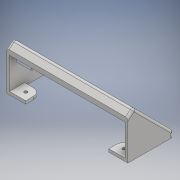
# Autodesk Inventor part: holder-LCD-screen
Saved by Autodesk Inventor 2018 (Build 220112000, 112)
## iProperties
Created: 2017-11-05
Part Number: holder-LCD-screen
Material: Generic
Document SubType Name: Modeling
Designer: Jurjen
Density: 1 g/cm^3
Appearance: Default
Author: Jurjen
Autodesk Inventor part; units mm, degrees
ref_plane "YZ Plane" through (0, 0, 0) normal (1, 0, 0) x (0, 1, 0)
ref_plane "XZ Plane" through (0, 0, 0) normal (0, 1, 0) x (-1, 0, 0)
ref_plane "XY Plane" through (0, 0, 0) normal (0, 0, 1) x (1, 0, 0)
sketch "Sketch1" plane through (0, 0, 0) normal (1, 0, 0) x (0, 1, 0)
  line L0 (-30, 25.7931) -> (-30, -25.7931)
  line L1 (30, -18.7931) -> (-21.6188, 32.8257)
  line L2 (-21.6188, 32.8257) -> (-30, 25.7931)
  line L3 (30, -18.7931) -> (30, -25.7931)
  line L4 (30, -25.7931) -> (-30, -25.7931)
  point P0 (0, 0)
  point P1 (-30, 0)
  point P2 (0, -25.7931)
  point P3 (-30, 0)
  dimension "d3" = 50
  dimension "d4" = 73
  dimension "d8" = 60
  dimension "d9" = 45
  dimension "d10" = 7
  constraints: 10 end point, 3 midpoint, 2 horizontal alignment, 2 vertical, 1 perpendicular, 1 vertical alignment
  measures "d3" angle of L2 L0
  measures "d4" distance of L1.start L1.end
  measures "d8" distance of L3.end L0.end
  measures "d9" angle of L4 L1
  measures "d10" distance of L1.start L3.end
extrude "Extrusion1" add sketch "Sketch1" along normal mid plane 160
sketch "Sketch2" plane through (-80, -21.6188, 32.8257) normal (0, 0.7071068, 0.7071068) x (1, 0, 0)
  line L0 (3.5, 69.5) -> (156.5, 69.5)
  line L1 (156.5, 69.5) -> (156.5, 3.5)
  line L2 (156.5, 3.5) -> (3.5, 3.5)
  line L3 (3.5, 3.5) -> (3.5, 69.5)
  line L4 (0, 0) -> (0, 73) projected
  line L5 (0, 0) -> (160, 0) projected
  line L6 (0, 73) -> (160, 73) projected
  line L7 (160, 73) -> (160, 0) projected
  point P0 (80, 38.4981)
  dimension "d11" = 3.5
  dimension "d12" = 3.5
  dimension "d13" = 3.5
  dimension "d14" = 3.5
  constraints: 8 end point, 2 parallel, 1 horizontal, 1 perpendicular
  measures "d11" distance between parallel lines of L4 L3
  measures "d12" distance between parallel lines of L5 L2
  measures "d13" distance between parallel lines of L6 L0
  measures "d14" distance between parallel lines of L7 L1
extrude "Extrusion2" cut sketch "Sketch2" against normal up to next contours L0 L1 L2 L3
sketch "Sketch3" plane through (-80, -21.6188, 32.8257) normal (0, 0.7071068, 0.7071068) x (1, 0, 0)
  line L0 (3.5, 3.5) -> (3.5, 69.5) projected
  line L1 (3.5, 69.5) -> (156.5, 69.5) projected
  line L2 (156.5, 69.5) -> (156.5, 3.5) projected
  line L3 (156.5, 3.5) -> (3.5, 3.5) projected
  line L4 (0, 0) -> (160, 0) projected
  line L5 (160, 73) -> (160, 0) projected
  line L6 (0, 73) -> (160, 73) projected
  line L7 (0, 0) -> (0, 73) projected
  line L8 (3.5, 69.5) -> (156.5, 69.5)
  line L9 (156.5, 69.5) -> (156.5, 3.5)
  line L10 (156.5, 3.5) -> (3.5, 3.5)
  line L11 (3.5, 3.5) -> (3.5, 69.5)
  line L12 (18.7, 55) -> (117.2, 55)
  line L13 (117.2, 55) -> (117.2, 14.5)
  line L14 (117.2, 14.5) -> (18.7, 14.5)
  line L15 (18.7, 14.5) -> (18.7, 55)
  circle A0 centre (143.6, 37.2) radius 6.25
  circle A1 centre (143.1, 56.2) radius 6.5
  point P0 (80, 38.4981)
  dimension "d17" = 98.5
  dimension "d18" = 40.5
  dimension "d19" = 26.4
  dimension "d20" = 12.5
  dimension "d21" = 22.7
  dimension "d22" = 15.2
  dimension "d23" = 11
  dimension "d67" = 13
  dimension "d69" = 0.5
  dimension "d70" = 19
  constraints: 16 end point, 4 parallel, 2 centre point, 2 horizontal, 2 perpendicular
  measures "d17" distance between parallel lines of L13 L15
  measures "d18" distance between parallel lines of L14 L12
  measures "d19" distance from line of L13 A0.centre
  measures "d20" diameter of A0
  measures "d21" distance from line of A0.centre L14
  measures "d22" distance between parallel lines of L0 L15
  measures "d23" distance between parallel lines of L3 L14
  measures "d67" diameter of A1
  measures "d69" horizontal distance of A0.centre A1.centre
  measures "d70" vertical distance of A0.centre A1.centre
extrude "Extrusion3" add sketch "Sketch3" against normal blind 3 contours L0 L1 L2 L3
fillet "Fillet1" radius 3 8 edges at (0, -21.6188, 32.8257) (-80, 4.1906, 7.0163) (-80, -25.8094, 29.3094) (80, -25.8094, 29.3094) (80, 4.1906, 7.0163) (0, 30, -18.7931) (-80, 30, -22.2931) (80, 30, -22.2931)
sketch "Sketch4" plane through (76.5, 18.0503, -25.7931) normal (0, 0, -1) x (-1, 0, 0)
  line L0 (137.8, -2.8995) -> (137.8, -31.5373) projected
  line L1 (137.8, -31.5373) -> (39.3, -31.5373) projected
  line L2 (39.3, -31.5373) -> (39.3, -2.8995) projected
  line L3 (39.3, -2.8995) -> (137.8, -2.8995) projected
  ellipse E0 centre (12.9, -15.486) end of major axis (19.15, -15.486) minor radius 4.4194 projected
  line L4 (153, 7.3536) -> (153, -39.3155) projected
  line L5 (0, 7.3536) -> (153, 7.3536) projected
  line L6 (0, -39.3155) -> (0, 7.3536) projected
  line L7 (153, -39.3155) -> (0, -39.3155) projected
  line L8 (153, 0) -> (153, -48.0503) projected
  line L9 (0, 7.3536) -> (153, 7.3536)
  line L10 (153, 7.3536) -> (153, 0)
  line L11 (153, 0) -> (0, 0)
  line L12 (0, 0) -> (0, 7.3536)
  point P0 (76.5, -18.0503)
  constraints: 8 end point, 2 parallel, 1 horizontal, 1 perpendicular, 1 other
extrude "Extrusion4" cut sketch "Sketch4" against normal up to next contours L4 L11 L6 L5
sketch "Sketch5" plane through (-80, 0, 0) normal (-1, 0, 0) x (0, 0, 1)
  line L0 (-13.3123, -0.2295) -> (7.9009, -21.4427)
  line L1 (7.9009, -21.4427) -> (12.1436, -17.2001)
  line L2 (12.1436, -17.2001) -> (-9.0696, 4.0131)
  line L3 (-9.0696, 4.0131) -> (-13.3123, -0.2295)
  line L4 (-20.0357, 27) -> (28.7606, -21.7963) projected
  line L5 (28.2295, -21.2652) -> (-18.4395, 25.4038) projected
  line L6 (-18.4395, 25.4038) -> (28.2295, -21.2652) projected
  line L7 (8.8195, -1.8552) -> (-0.0194, 6.9837) projected
  line L8 (-8.1865, 15.1508) -> (20.4514, -13.4871) projected
  line L9 (20.4514, -13.4871) -> (-8.1865, 15.1508) projected
  point P0 (0, 0)
  dimension "d35" = 30
  dimension "d36" = 6
  dimension "d39" = 14.5
  dimension "d40" = 15
  constraints: 8 end point, 3 perpendicular, 1 parallel
  measures "d35" distance of L1.end L2.end
  measures "d36" distance between parallel lines of L2 L0
  measures "d39" distance between parallel lines of L4 L0
  measures "d40" distance from line of L4.end L1
extrude "Extrusion5" cut sketch "Sketch5" against normal up to next
sketch "Sketch6" plane through (-77, -19.675, 30.8819) normal (0, 0.7071068, 0.7071068) x (1, 0, 0)
  circle A0 centre (4.1, 61.451) radius 1.6
  circle A1 centre (4.1, 11.951) radius 1.6
  circle A2 centre (148.6, 61.451) radius 1.6
  circle A3 centre (148.6, 11.951) radius 1.6
  line L0 (0.5, 71.9508) -> (0.5, 32.7743) projected
  line L1 (0.5, 0.751) -> (153.5, 0.751) projected
  circle A4 centre (5.7, 61.451) radius 1.6
  circle A5 centre (5.7, 11.951) radius 1.6
  circle A6 centre (147, 11.951) radius 1.6
  circle A7 centre (147, 61.451) radius 1.6
  line L2 (147, 63.051) -> (148.6, 63.051)
  line L3 (147, 59.851) -> (148.6, 59.851)
  line L4 (4.1, 63.051) -> (5.7, 63.051)
  line L5 (4.1, 59.851) -> (5.7, 59.851)
  line L6 (4.1, 13.551) -> (5.7, 13.551)
  line L7 (5.7, 10.351) -> (4.1, 10.351)
  line L8 (147, 13.551) -> (148.6, 13.551)
  line L9 (147, 10.351) -> (148.6, 10.351)
  point P0 (77, 35.7491)
  dimension "d41" = 3.2
  dimension "d42" = 144.5
  dimension "d43" = 49.5
  dimension "d44" = 3.6
  dimension "d45" = 11.2
  constraints: 20 point on circle, 16 end point, 9 tangent, 8 centre point, 7 equal radius, 5 parallel, 3 point on line, 2 horizontal, 2 horizontal alignment, 2 vertical alignment
  measures "d41" diameter of A0
  measures "d42" distance of A2.centre A0.centre
  measures "d43" distance of A0.centre A1.centre
  measures "d44" distance from line of A0.centre L0
  measures "d45" distance from line of A1.centre L1
extrude "Extrusion6" cut sketch "Sketch6" against normal up to next contours A0 A4 | A0 A4 | A1 A5 | A1 A5 | A2 A7 | A2 A7 L2 | L3 A7 A2 | A7 A2 | A2 A7 | A3 A6 | A3 A6 L8 | L9 A6 A3 | A6 A3 | A3 A6 picked at (3.0447, 61.5129) picked at (4.6405, 61.451) picked at (3.0447, 12.0129) picked at (4.6405, 11.951)
chamfer "Chamfer1" distance 2 angle 45 4 edges at (-80, -10.8361, -2.7057) (-80, 1.8918, -11.191) (-80, -6.5935, 1.537) (-80, -19.3214, 10.0222)
sketch "Sketch7" plane through (77, 30, -25.7931) normal (0, 0, -1) x (-1, 0, 0)
  line L0 (157, -51.7963) -> (157, -60) projected
  line L1 (157, -60) -> (132, -60)
  line L2 (132, -60) -> (132, -40)
  line L3 (132, -40) -> (157, -40)
  line L4 (157, -40) -> (157, -60)
  point P0 (77, -30)
  dimension "d51" = 25
  dimension "d52" = 20
  constraints: 8 end point, 2 parallel, 1 horizontal, 1 perpendicular
  measures "d51" distance between parallel lines of L4 L2
  measures "d52" distance between parallel lines of L1 L3
extrude "Extrusion7" add sketch "Sketch7" against normal blind 4
sketch "Sketch8" plane through (77, 30, -25.7931) normal (0, 0, -1) x (-1, 0, 0)
  circle A0 centre (142, -50) radius 2.1
  line L0 (157, -60) -> (132, -60) projected
  line L1 (132, -60) -> (132, -40) projected
  point P0 (77, -30)
  dimension "d55" = 10
  dimension "d56" = 10
  dimension "d57" = 4.2
  constraints: 1 centre point
  measures "d55" distance from line of L0 A0.centre
  measures "d56" distance from line of L1 A0.centre
  measures "d57" diameter of A0
fillet "Fillet2" radius 10 1 edges at (-55, -10, -23.7931)
extrude "Extrusion8" cut sketch "Sketch8" against normal up to next
mirror "Mirror1" about plane through (0, 0, 0) normal (1, 0, 0) of "Extrusion7", "Fillet2", "Extrusion8"
sketch "Sketch9" plane through (-77, -19.675, 30.8819) normal (0, 0.7071068, 0.7071068) x (1, 0, 0)
  line L0 (15.7, 64.6999) -> (54.0715, 64.6999) construction
  line L1 (54.0715, 64.6999) -> (54.0715, 56.5594) construction
  line L2 (54.0715, 56.5594) -> (15.7, 56.5594) construction
  line L3 (15.7, 56.5594) -> (15.7, 64.6999) construction
  line L4 (15.7, 52.251) -> (114.2, 52.251) projected
  line L5 (0, 69.0084) -> (154, 69.0084) projected
  line L6 (114.2, 52.251) -> (114.2, 69.0084) construction
  line L7 (21.5476, 60.6463) -> (20.0354, 60.3719)
  spline S0 degree 2 poles (20.0354, 60.3719) (19.9622, 60.8231) (19.4195, 61.2804) (18.9866, 61.2804) knots 0 0 0 1 2 2 2
  spline S1 degree 2 poles (18.9866, 61.2804) (18.4195, 61.2804) (17.7366, 60.4877) (17.7366, 59.5609) knots 0 0 0 1 2 2 2
  spline S2 degree 2 poles (17.7366, 59.5609) (17.7366, 58.5304) (18.4317, 57.6829) (19.011, 57.6829) knots 0 0 0 1 2 2 2
  spline S3 degree 2 poles (19.011, 57.6829) (19.45, 57.6829) (20.0049, 58.1829) (20.1207, 58.7865) knots 0 0 0 1 2 2 2
  line L8 (20.1207, 58.7865) -> (21.6268, 58.5304)
  spline S4 degree 2 poles (21.6268, 58.5304) (21.3951, 57.4938) (20.0598, 56.4329) (18.9439, 56.4329) knots 0 0 0 1 2 2 2
  spline S5 degree 2 poles (18.9439, 56.4329) (17.6756, 56.4329) (16.1634, 58.0365) (16.1634, 59.4572) knots 0 0 0 1 2 2 2
  spline S6 degree 2 poles (16.1634, 59.4572) (16.1634, 60.8902) (17.6756, 62.4877) (18.9683, 62.4877) knots 0 0 0 1 2 2 2
  spline S7 degree 2 poles (18.9683, 62.4877) (20.0293, 62.4877) (21.2732, 61.5792) (21.5476, 60.6463) knots 0 0 0 1 2 2 2
  spline S8 degree 2 poles (22.3585, 59.5426) (22.3585, 60.3048) (23.1146, 61.7377) (24.4927, 62.4877) (25.3463, 62.4877) knots 0 0 0 1 2 3 3 3
  spline S9 degree 2 poles (25.3463, 62.4877) (26.6634, 62.4877) (28.3463, 60.7804) (28.3463, 59.4755) knots 0 0 0 1 2 2 2
  spline S10 degree 2 poles (28.3463, 59.4755) (28.3463, 58.1646) (26.6451, 56.4329) (25.3585, 56.4329) knots 0 0 0 1 2 2 2
  spline S11 degree 2 poles (25.3585, 56.4329) (24.5598, 56.4329) (23.1146, 57.1524) (22.3585, 58.5426) (22.3585, 59.5426) knots 0 0 0 1 2 3 3 3
  spline S12 degree 2 poles (23.9317, 59.4633) (23.9317, 58.5975) (24.7488, 57.6829) (25.3524, 57.6829) knots 0 0 0 1 2 2 2
  spline S13 degree 2 poles (25.3524, 57.6829) (25.9561, 57.6829) (26.7671, 58.5975) (26.7671, 59.4694) knots 0 0 0 1 2 2 2
  spline S14 degree 2 poles (26.7671, 59.4694) (26.7671, 60.3231) (25.9561, 61.2377) (25.3524, 61.2377) knots 0 0 0 1 2 2 2
  spline S15 degree 2 poles (25.3524, 61.2377) (24.7488, 61.2377) (23.9317, 60.3231) (23.9317, 59.4633) knots 0 0 0 1 2 2 2
  line L9 (31.0171, 56.5609) -> (29.4805, 56.5609)
  line L10 (29.4805, 56.5609) -> (29.4805, 62.3597)
  line L11 (29.4805, 62.3597) -> (30.9073, 62.3597)
  line L12 (30.9073, 62.3597) -> (30.9073, 61.5365)
  spline S16 degree 2 poles (30.9073, 61.5365) (31.2732, 62.1219) (31.8524, 62.4877) (32.2244, 62.4877) knots 0 0 0 1 2 2 2
  spline S17 degree 2 poles (32.2244, 62.4877) (32.7488, 62.4877) (33.2305, 62.1951) knots 0 0 0 1 1 1
  line L13 (33.2305, 62.1951) -> (32.761, 60.8597)
  spline S18 degree 2 poles (32.761, 60.8597) (32.3707, 61.1097) (32.0415, 61.1097) knots 0 0 0 1 1 1
  spline S19 degree 2 poles (32.0415, 61.1097) (31.7183, 61.1097) (31.2732, 60.756) (31.0171, 59.8292) (31.0171, 58.3475) knots 0 0 0 1 2 3 3 3
  line L14 (31.0171, 58.3475) -> (31.0171, 56.5609)
  line L15 (37.2488, 58.4085) -> (38.7793, 58.1524)
  spline S20 degree 2 poles (38.7793, 58.1524) (38.4866, 57.3109) (37.2122, 56.4329) (36.2549, 56.4329) knots 0 0 0 1 2 2 2
  spline S21 degree 2 poles (36.2549, 56.4329) (34.7427, 56.4329) (34.0171, 57.4207) knots 0 0 0 1 1 1
  spline S22 degree 2 poles (34.0171, 57.4207) (33.4439, 58.2133) (33.4439, 59.4146) knots 0 0 0 1 1 1
  spline S23 degree 2 poles (33.4439, 59.4146) (33.4439, 60.8597) (34.95, 62.4877) (36.1024, 62.4877) knots 0 0 0 1 2 2 2
  spline S24 degree 2 poles (36.1024, 62.4877) (37.3951, 62.4877) (38.889, 60.7804) (38.8585, 59.0182) knots 0 0 0 1 2 2 2
  line L16 (38.8585, 59.0182) -> (35.0171, 59.0182)
  spline S25 degree 2 poles (35.0171, 59.0182) (35.0354, 58.3353) (35.7427, 57.5792) (36.2732, 57.5792) knots 0 0 0 1 2 2 2
  spline S26 degree 2 poles (36.2732, 57.5792) (36.6329, 57.5792) (37.1207, 57.9694) (37.2488, 58.4085) knots 0 0 0 1 2 2 2
  spline S27 degree 2 poles (37.3341, 59.9572) (37.3159, 60.6219) (36.6634, 61.317) (36.1939, 61.317) knots 0 0 0 1 2 2 2
  spline S28 degree 2 poles (36.1939, 61.317) (35.6939, 61.317) (35.3646, 60.9511) knots 0 0 0 1 1 1
  spline S29 degree 2 poles (35.3646, 60.9511) (35.0415, 60.5853) (35.0415, 59.9572) knots 0 0 0 1 1 1
  line L17 (35.0415, 59.9572) -> (37.3341, 59.9572)
  line L18 (42.258, 60.8592) -> (39.8018, 64.6999)
  line L19 (39.8018, 64.6999) -> (41.169, 64.6999)
  line L20 (41.169, 64.6999) -> (42.9184, 61.8382)
  line L21 (42.9184, 61.8382) -> (44.6679, 64.6999)
  line L22 (44.6679, 64.6999) -> (46.0408, 64.6999)
  line L23 (46.0408, 64.6999) -> (43.5846, 60.8592)
  line L24 (43.5846, 60.8592) -> (46.2667, 56.6999)
  line L25 (46.2667, 56.6999) -> (44.8996, 56.6999)
  line L26 (44.8996, 56.6999) -> (42.9184, 59.8802)
  line L27 (42.9184, 59.8802) -> (40.9431, 56.6999)
  line L28 (40.9431, 56.6999) -> (39.5759, 56.6999)
  line L29 (39.5759, 56.6999) -> (42.258, 60.8592)
  line L30 (46.539, 64.6999) -> (47.8134, 64.6999)
  line L31 (47.8134, 64.6999) -> (49.9742, 61.1547)
  line L32 (49.9742, 61.1547) -> (52.1291, 64.6999)
  line L33 (52.1291, 64.6999) -> (53.4094, 64.6999)
  line L34 (53.4094, 64.6999) -> (50.6346, 60.2336)
  line L35 (50.6346, 60.2336) -> (50.6346, 56.6999)
  line L36 (50.6346, 56.6999) -> (49.3543, 56.6999)
  line L37 (49.3543, 56.6999) -> (49.3543, 60.2336)
  line L38 (49.3543, 60.2336) -> (46.539, 64.6999)
  point P0 (77, 35.7491)
  point P1 (114.2, 60.6297)
  point P2 (15.7, 60.6297)
  constraints: 2 end point, 2 midpoint, 1 horizontal alignment, 1 point on line, 1 vertical, 1 vertical alignment, 2 other
emboss "Emboss1" sketch "Sketch9" operation cut depth 1 direction (0, -0.7071068, -0.7071068)
sketch "Sketch10" plane through (80, 0, 0) normal (1, 0, 0) x (0, 0, -1)
  line L0 (-28.7606, -21.7963) -> (20.0357, 27) projected
  line L1 (25.7931, 30) -> (20.0357, 30) projected
  line L2 (-31.0587, -23.7246) -> (-25.7931, -30) projected
  line L3 (20.0357, 27) -> (-28.7606, -21.7963)
  line L4 (-28.7606, -21.7963) -> (-30.8819, -19.675) projected
  line L5 (-28.7606, -21.7963) -> (-30.89, -23.9257)
  line L6 (-25.7931, -30) -> (-31.0587, -23.7246) projected
  line L7 (20.0357, 27) -> (23.0357, 30)
  line L8 (-30.89, -23.9257) -> (-32.8584, -45.343)
  line L9 (-32.8584, -45.343) -> (26.976, -47.0964)
  line L10 (26.976, -47.0964) -> (26.976, 43.6415)
  line L11 (26.976, 43.6415) -> (23.0357, 30)
  point P0 (0, 0)
  constraints: 14 end point, 2 collinear, 2 point on line, 1 vertical
sketch "Sketch11" plane through (-77, -19.675, 30.8819) normal (0, 0.7071068, 0.7071068) x (1, 0, 0)
  line L0 (-12.1543, 90.1766) -> (102.3772, 90.1766)
  line L1 (102.3772, 90.1766) -> (102.3772, -17.0089)
  line L2 (102.3772, -17.0089) -> (-12.1543, -17.0089)
  line L3 (-12.1543, -17.0089) -> (-12.1543, 90.1766)
  point P0 (77, 35.7491)
  constraints: 8 end point, 2 parallel, 1 horizontal, 1 perpendicular
equation "\"d12\" = d11"
equation "\"d13\" = d11"
equation "\"d14\" = d11"
body "Solid1"
